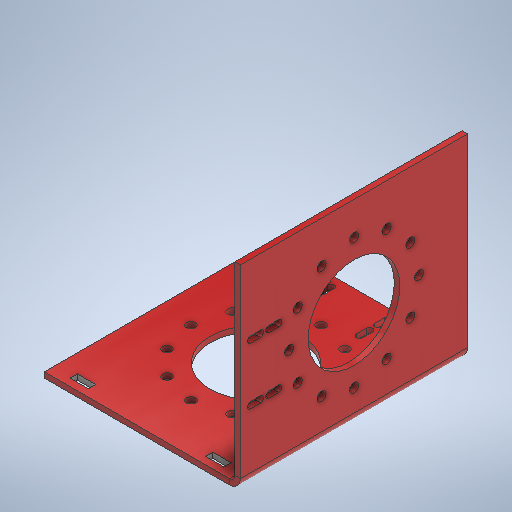
# Autodesk Inventor part: Face with Harmonic Drive
Saved by Autodesk Inventor 2025 (Build 290162000, 162)
## iProperties
Created: 2025-08-10
Part Number: Face with Harmonic Drive
Material: Steel, Carbon
Document SubType Name: Sheet Metal
Designer: yshis
Density: 7.85 g/cm^3
Sheet Metal Rule: Default
Appearance: Semi-Polished
Author: yshis
Autodesk Inventor part; units mm, degrees
ref_plane "YZ Plane" through (0, 0, 0) normal (1, 0, 0) x (0, 1, 0)
ref_plane "XZ Plane" through (0, 0, 0) normal (0, 1, 0) x (-1, 0, 0)
ref_plane "XY Plane" through (0, 0, 0) normal (0, 0, 1) x (1, 0, 0)
sketch "Sketch1" plane through (0, 0, 0) normal (0, 1, 0) x (-1, 0, 0)
  line L0 (0, 0) -> (107, 0)
  line L1 (107, 0) -> (107, -124)
  line L2 (107, -124) -> (0, -124)
  line L3 (0, -124) -> (0, 0)
  circle A0 centre (53.5, -62) radius 25
  circle A1 centre (18, -62) radius 2.5
  circle A2 centre (22.7561, -79.75) radius 2.5
  circle A3 centre (35.75, -92.7439) radius 2.5
  circle A4 centre (53.5, -97.5) radius 2.5
  circle A5 centre (71.25, -92.7439) radius 2.5
  circle A6 centre (84.2439, -79.75) radius 2.5
  circle A7 centre (89, -62) radius 2.5
  circle A8 centre (84.2439, -44.25) radius 2.5
  circle A9 centre (71.25, -31.2561) radius 2.5
  circle A10 centre (53.5, -26.5) radius 2.5
  circle A11 centre (35.75, -31.2561) radius 2.5
  circle A12 centre (22.7561, -44.25) radius 2.5
  line L4 (69, -111.25) -> (69, -111.25)
  line L5 (67.25, -113) -> (67.25, -118.5)
  line L6 (69, -120.25) -> (69, -120.25)
  line L7 (70.75, -118.5) -> (70.75, -113)
  arc A13 (69, -120.25) -> (70.75, -118.5) centre (69, -118.5) ccw
  arc A14 (67.25, -118.5) -> (69, -120.25) centre (69, -118.5) ccw
  arc A15 (69, -111.25) -> (67.25, -113) centre (69, -113) ccw
  arc A16 (70.75, -113) -> (69, -111.25) centre (69, -113) ccw
  line L8 (38, -111.25) -> (38, -111.25)
  arc A17 (38, -111.25) -> (36.25, -113) centre (38, -113) ccw
  arc A18 (39.75, -113) -> (38, -111.25) centre (38, -113) ccw
  line L9 (36.25, -113) -> (36.25, -118.5)
  line L10 (39.75, -118.5) -> (39.75, -113)
  line L11 (38, -120.25) -> (38, -120.25)
  arc A19 (36.25, -118.5) -> (38, -120.25) centre (38, -118.5) ccw
  arc A20 (38, -120.25) -> (39.75, -118.5) centre (38, -118.5) ccw
  line L12 (69, -101.25) -> (69, -101.25)
  arc A21 (69, -101.25) -> (67.25, -103) centre (69, -103) ccw
  arc A22 (70.75, -103) -> (69, -101.25) centre (69, -103) ccw
  line L13 (67.25, -103) -> (67.25, -108.5)
  line L14 (70.75, -108.5) -> (70.75, -103)
  line L15 (69, -110.25) -> (69, -110.25)
  arc A23 (67.25, -108.5) -> (69, -110.25) centre (69, -108.5) ccw
  arc A24 (69, -110.25) -> (70.75, -108.5) centre (69, -108.5) ccw
  line L16 (38, -101.25) -> (38, -101.25)
  arc A25 (38, -101.25) -> (36.25, -103) centre (38, -103) ccw
  arc A26 (39.75, -103) -> (38, -101.25) centre (38, -103) ccw
  line L17 (36.25, -103) -> (36.25, -108.5)
  line L18 (39.75, -108.5) -> (39.75, -103)
  line L19 (38, -110.25) -> (38, -110.25)
  arc A27 (36.25, -108.5) -> (38, -110.25) centre (38, -108.5) ccw
  arc A28 (38, -110.25) -> (39.75, -108.5) centre (38, -108.5) ccw
  point P0 (70.75, -115.75)
  point P1 (53.5, -124)
  point P2 (39.75, -115.75)
  point P3 (70.75, -105.75)
  point P4 (39.75, -105.75)
  point P5 (38, -101.25)
  point P6 (38, -110.25)
  point P7 (69, -101.25)
  point P8 (69, -110.25)
  point P9 (38, -111.25)
  point P10 (38, -120.25)
  point P11 (69, -111.25)
  point P12 (69, -120.25)
  dimension "d0" = 107
  dimension "d1" = 124
  dimension "d2" = 50
  dimension "d3" = 62
  dimension "d4" = 53.5
  dimension "d5" = 5
  dimension "d6" = 35.5
  dimension "d9" = 360
  dimension "d11" = 3.5
  dimension "d12" = 9
  dimension "d13" = 1.75
  dimension "d14" = 15.5
  dimension "d15" = 56.5
  dimension "d18" = 31
  dimension "d21" = 10
  measures "d0" distance of L1.end L2.end
  measures "d1" distance of L0.end L1.end
  measures "d2" diameter of A0
  measures "d3" distance from line of A0.centre L0
  measures "d4" distance from line of A0.centre L3
  measures "d5" diameter of A1
  measures "d6" distance of A1.centre A0.centre
  measures "d11" distance from line of L5 point (70.75, -115.75)
  measures "d12" distance between parallel lines of L6 L4
  measures "d13" radius of A13
  measures "d14" horizontal distance of A13.centre point (53.5, -124)
  measures "d15" vertical distance of A13.centre A0.centre
  measures "d18" distance of L4.start L8.start
  measures "d21" distance of L4.start L12.start
extrude "Plate1" add sketch "Sketch1" along normal blind 3
sketch "Sketch2" plane through (-3, 0, -124) normal (1, 0, 0) x (0, 1, 0)
  line L0 (0, 124) -> (0, 0)
  line L1 (0, 0) -> (107, 0)
  line L2 (107, 0) -> (107, 124)
  line L3 (107, 124) -> (0, 124)
  constraints: 6 end point, 1 horizontal, 1 perpendicular, 1 vertical
edge flange "Flange1" height 107 angle 90 thickness 3 bend radius 3 thickness toward (1, 0, 0) relief straight relief width 3 relief depth 1.5 edges at (0, 3, -62) wall of the first edge with corners at (-3, 0, 0) (-3, 0, -124) (-3, 107, -124) (-3, 107, 0)
bend "Bend1"
corner "Corner1"
sketch "Sketch3" plane through (0, 107, 0) normal (1, 0, 0) x (0, 0, -1)
  circle A0 centre (62, -53.5) radius 25
  line L0 (0, 0) -> (124, 0) projected
  line L1 (124, 0) -> (124, -101) projected
  circle A1 centre (62, -18) radius 2.5
  circle A2 centre (44.25, -22.7561) radius 2.5
  circle A3 centre (31.2561, -35.75) radius 2.5
  circle A4 centre (26.5, -53.5) radius 2.5
  circle A5 centre (31.2561, -71.25) radius 2.5
  circle A6 centre (44.25, -84.2439) radius 2.5
  circle A7 centre (62, -89) radius 2.5
  circle A8 centre (79.75, -84.2439) radius 2.5
  circle A9 centre (92.7439, -71.25) radius 2.5
  circle A10 centre (97.5, -53.5) radius 2.5
  circle A11 centre (92.7439, -35.75) radius 2.5
  circle A12 centre (79.75, -22.7561) radius 2.5
  line L2 (11, -70.75) -> (5.5, -70.75)
  line L3 (3.75, -69) -> (3.75, -69)
  line L4 (5.5, -67.25) -> (11, -67.25)
  line L5 (12.75, -69) -> (12.75, -69)
  arc A13 (3.75, -69) -> (5.5, -70.75) centre (5.5, -69) ccw
  arc A14 (5.5, -67.25) -> (3.75, -69) centre (5.5, -69) ccw
  arc A15 (12.75, -69) -> (11, -67.25) centre (11, -69) ccw
  arc A16 (11, -70.75) -> (12.75, -69) centre (11, -69) ccw
  line L6 (12.75, -38) -> (12.75, -38)
  arc A17 (12.75, -38) -> (11, -36.25) centre (11, -38) ccw
  arc A18 (11, -39.75) -> (12.75, -38) centre (11, -38) ccw
  line L7 (5.5, -36.25) -> (11, -36.25)
  line L8 (11, -39.75) -> (5.5, -39.75)
  line L9 (3.75, -38) -> (3.75, -38)
  arc A19 (3.75, -38) -> (5.5, -39.75) centre (5.5, -38) ccw
  arc A20 (5.5, -36.25) -> (3.75, -38) centre (5.5, -38) ccw
  line L10 (22.75, -69) -> (22.75, -69)
  arc A21 (22.75, -69) -> (21, -67.25) centre (21, -69) ccw
  arc A22 (21, -70.75) -> (22.75, -69) centre (21, -69) ccw
  line L11 (15.5, -67.25) -> (21, -67.25)
  line L12 (21, -70.75) -> (15.5, -70.75)
  line L13 (13.75, -69) -> (13.75, -69)
  arc A23 (13.75, -69) -> (15.5, -70.75) centre (15.5, -69) ccw
  arc A24 (15.5, -67.25) -> (13.75, -69) centre (15.5, -69) ccw
  line L14 (22.75, -38) -> (22.75, -38)
  arc A25 (22.75, -38) -> (21, -36.25) centre (21, -38) ccw
  arc A26 (21, -39.75) -> (22.75, -38) centre (21, -38) ccw
  line L15 (15.5, -36.25) -> (21, -36.25)
  line L16 (21, -39.75) -> (15.5, -39.75)
  line L17 (13.75, -38) -> (13.75, -38)
  arc A27 (13.75, -38) -> (15.5, -39.75) centre (15.5, -38) ccw
  arc A28 (15.5, -36.25) -> (13.75, -38) centre (15.5, -38) ccw
  point P0 (0, -107)
  point P1 (62, 0)
  point P2 (12.75, -70.75)
  point P3 (3.75, -70.75)
  point P4 (12.75, -67.25)
  point P5 (12.75, -36.25)
  point P6 (12.75, -39.75)
  point P7 (3.75, -39.75)
  point P8 (22.75, -67.25)
  point P9 (22.75, -70.75)
  point P10 (13.75, -70.75)
  point P11 (22.75, -36.25)
  point P12 (22.75, -39.75)
  point P13 (13.75, -39.75)
  point P14 (13.75, -69)
  point P15 (12.75, -38)
  point P16 (3.75, -38)
  point P17 (12.75, -69)
  point P18 (3.75, -69)
  dimension "d35" = 50
  dimension "d36" = 53.5
  dimension "d37" = 62
  dimension "d38" = 5
  dimension "d39" = 35.5
  dimension "d42" = 360
  dimension "d44" = 3.5
  dimension "d45" = 9
  dimension "d46" = 1.75
  dimension "d47" = 15.5
  dimension "d48" = 56.5
  dimension "d51" = 31
  dimension "d54" = 10
  constraints: 32 end point, 32 point on circle, 29 centre point, 24 point on line, 8 tangent, 3 equal radius, 2 coincident, 2 horizontal, 2 parallel, 1 midpoint, 1 perpendicular, 1 vertical, 104 other
  measures "d35" diameter of A0
  measures "d36" distance of A0.centre point (62, 0)
  measures "d37" distance from line of A0.centre L1
  measures "d38" diameter of A1
  measures "d39" distance of A1.centre A0.centre
  measures "d44" distance of point (12.75, -67.25) point (12.75, -70.75)
  measures "d45" distance of point (12.75, -70.75) point (3.75, -70.75)
  measures "d46" radius of A13
  measures "d47" vertical distance of point (62, -53.5) A13.centre
  measures "d48" horizontal distance of A0.centre A13.centre
  measures "d51" distance of point (12.75, -67.25) point (12.75, -36.25)
  measures "d54" distance of point (12.75, -67.25) point (22.75, -67.25)
extrude "Cut1" cut sketch "Sketch3" against normal blind 3
sketch "Sketch4" plane through (0, 0, 0) normal (0, -1, 0) x (1, 0, 0)
  line L0 (-13, -4) -> (-23, -4)
  line L1 (-23, -4) -> (-23, -8)
  line L2 (-23, -8) -> (-13, -8)
  line L3 (-13, -8) -> (-13, -4)
  line L4 (-107, 0) -> (-6, 0) projected
  line L5 (0, 0) -> (0, -124) projected
  line L6 (-87, -4) -> (-97, -4)
  line L7 (-97, -4) -> (-97, -8)
  line L8 (-97, -8) -> (-87, -8)
  line L9 (-87, -8) -> (-87, -4)
  line L10 (-13, -116) -> (-23, -116)
  line L11 (-23, -116) -> (-23, -120)
  line L12 (-23, -120) -> (-13, -120)
  line L13 (-13, -120) -> (-13, -116)
  line L14 (-87, -116) -> (-97, -116)
  line L15 (-97, -116) -> (-97, -120)
  line L16 (-97, -120) -> (-87, -120)
  line L17 (-87, -120) -> (-87, -116)
  dimension "d59" = 10
  dimension "d60" = 4
  dimension "d61" = 4
  dimension "d62" = 13
  dimension "d65" = 74
  dimension "d68" = 112
  constraints: 32 end point, 2 horizontal, 2 parallel, 1 perpendicular, 1 vertical, 24 other
  measures "d59" distance of L1.end L2.end
  measures "d60" distance of L0.end L1.end
  measures "d61" distance between parallel lines of L4 L0
  measures "d62" distance between parallel lines of L5 L3
  measures "d65" distance of L0.start L6.start
  measures "d68" distance of L0.start L10.start
extrude "Cut2" cut sketch "Sketch4" against normal blind 3
unfold all bends "Unfold1" k factor 0.44 fixed face at (-101.8333, 3, -62)
refold all bends "Refold1"
equation "\"d36\" = d4"
equation "\"d45\" = d12"
equation "\"d47\" = d14"
equation "\"d51\" = d18"
equation "\"d54\" = d21"
equation "\"d3\" = 0.5 * d1"
equation "\"d4\" = 0.5 * d0"
equation "\"d13\" = 0.5 * d11"
equation "\"d18\" = 2 * d14"
equation "\"d37\" = d3"
equation "\"d39\" = d6"
equation "\"d48\" = d15"
equation "\"d57\" = Thickness"
equation "\"d68\" = d1 - d60 - 2 * d61"
equation "\"d71\" = Thickness"
equation "\"d24\" = Thickness"
equation "\"d25\" = BendReliefWidth"
equation "\"d26\" = BendReliefDepth"
equation "\"d27\" = MinimumRemnant"
equation "\"d28\" = TransitionRadius"
equation "\"d29\" = d0"
equation "\"d31\" = BendRadius"
equation "\"d32\" = CornerReliefSize"
equation "\"d33\" = GapSize"
equation "\"d34\" = JacobiRadiusSize"
equation "\"BendRadius\" = Thickness"
equation "\"BendReliefWidth\" = Thickness"
equation "\"BendReliefDepth\" = 0.5 * Thickness"
equation "\"CornerReliefSize\" = 4 * Thickness"
equation "\"MinimumRemnant\" = 2 * Thickness"
equation "\"TransitionRadius\" = BendRadius"
equation "\"JacobiRadiusSize\" = BendRadius"
equation "\"GapSize\" = Thickness"
equation "\"Thickness\" = 3"
body "Solid1"
